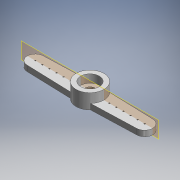
# Autodesk Inventor part: SG90Horn2
Saved by Autodesk Inventor 2019.2 (Build 232265000, 265)
## iProperties
Part Number: SG90Horn2
Material: PC/ABS Plastic
Document SubType Name: Modeling
Designer: richard.girt
Mass: 0.0812789 g
Surface Area: 4.79705 cm^2
Volume: 0.227498 cm^3
Density: 0.357273 g/cm^3
Appearance: Smooth - White
Author: richard.girt
Autodesk Inventor part; units mm, degrees
ref_plane "YZ Plane" through (0, 0, 0) normal (1, 0, 0) x (0, 1, 0)
ref_plane "XZ Plane" through (0, 0, 0) normal (0, 1, 0) x (-1, 0, 0)
sketch "Sketch1" plane through (0, 0, 0) normal (0, 1, 0) x (-1, 0, 0)
  circle A0 centre (0, 0) radius 3.45
  line L0 (0, 0) -> (-13.55, 0) construction
  line L1 (-0.0814, 2.4486) -> (-13.6164, 1.9989)
  line L2 (-13.6164, -1.9989) -> (-0.0814, -2.4486)
  arc A1 (-0.0814, -2.4486) -> (-0.0814, 2.4486) centre (0, 0) ccw
  arc A2 (-13.6164, 1.9989) -> (-13.6164, -1.9989) centre (-13.55, 0) ccw
  point P0 (-6.775, 0)
  point P1 (-15.55, 0)
  point P2 (3.45, 0)
  dimension "d0" = 6.9
  dimension "d2" = 4
  dimension "d3" = 1
  dimension "d4" = 19
  constraints: 8 end point, 5 point on circle, 4 tangent, 2 centre point, 2 horizontal alignment, 1 coincident, 1 horizontal, 1 midpoint, 2 other
  measures "d2" diameter of A2
  measures "d4" distance of point (-15.55, 0) point (3.45, 0)
extrude "Extrusion1" add sketch "Sketch1" along normal blind 1.4
extrude "Extrusion2" add sketch "Sketch1" along normal blind 3.7 contours A0 L2 A1 L1 | L1 A1 L2 A0
sketch "Sketch2" plane through (0, 3.7, 0) normal (0, 1, 0) x (1, 0, 0)
  circle A0 centre (0, 0) radius 3.45 construction
  circle A1 centre (0, 0) radius 1.2
  dimension "d9" = 2.4
  constraints: 1 centre point, 1 coincident
  measures "d9" diameter of A1
extrude "Extrusion3" cut sketch "Sketch2" against normal through all
sketch "Sketch3" plane through (0, 3.7, 0) normal (0, 1, 0) x (1, 0, 0)
  circle A0 centre (0, 0) radius 3.45 construction
  circle A1 centre (0, 0) radius 2.3
  dimension "d12" = 4.6
  constraints: 1 centre point, 1 coincident
  measures "d12" diameter of A1
extrude "Extrusion4" cut sketch "Sketch3" against normal blind 2
sketch "Sketch4" plane through (0, 0, 0) normal (0, -1, 0) x (1, 0, 0)
  arc A0 (2.509, 2.368) -> (2.509, -2.368) centre (0, 0) ccw construction
  circle A1 centre (0, 0) radius 2.35
  dimension "d15" = 1.1
  constraints: 1 centre point, 1 coincident
  measures "d15" radial gap between concentric circles of A0 A1
extrude "Extrusion5" cut sketch "Sketch4" against normal blind 1
sketch "Sketch5" plane through (0, 0, 0) normal (0, -1, 0) x (1, 0, 0)
  arc A0 (13.6164, -1.9989) -> (13.6164, 1.9989) centre (13.55, 0) ccw construction
  line L0 (13.55, 0) -> (10.05, 0)
  line L1 (10.05, 0) -> (6.55, 0)
  line L2 (6.55, 0) -> (3.05, 0)
  point P0 (8.3, 0)
  point P1 (4.8, 0)
  point P2 (11.8, 0)
  point P3 (4.8, 0)
  dimension "d18" = 3.5
  constraints: 6 end point, 4 coincident, 3 midpoint, 2 collinear, 2 horizontal, 1 point on line
  measures "d18" distance of L0.start L0.end
hole "Hole1" at (13.55, 0, 0) at (10.05, 0, 0) at (8.3, 0, 0) at (6.55, 0, 0) at (4.8, 0, 0) at (11.8, 0, 0) direction (0, 1, 0) diameter 0.3 end through all
mirror "Mirror1" about plane through (0, 0, 0) normal (1, 0, 0)
body "Solid1"
